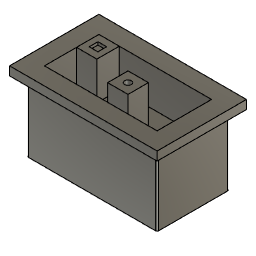
Button_Body (Autodesk Fusion 360 design; units mm, degrees)
Autodesk Fusion 360 part; units mm, degrees
sketch "Sketch1" plane through (0, 0, 0) normal (0, 0, 1) x (1, 0, 0)
  line L0 (0.5, 0) -> (44.2, 0)
  line L1 (44.7, 0.5) -> (44.7, 24.2)
  line L2 (44.2, 24.7) -> (0.5, 24.7)
  line L3 (44.7, 24.7) -> (0, 0) construction
  line L4 (0, 24.7) -> (44.7, 0) construction
  arc A0 (0.5, 24.7) -> (0, 24.2) centre (0.5, 24.2) ccw
  arc A1 (0, 0.5) -> (0.5, 0) centre (0.5, 0.5) ccw
  arc A2 (44.2, 0) -> (44.7, 0.5) centre (44.2, 0.5) ccw
  arc A3 (44.7, 24.2) -> (44.2, 24.7) centre (44.2, 24.2) ccw
  line L5 (22.35, 12.35) -> (22.35, 24.7) construction
  line L6 (22.35, 12.35) -> (0, 12.35) construction
  line L7 (22.35, 12.35) -> (22.35, 0) construction
  circle A4 centre (39.7, 12.35) radius 1.35
  circle A5 centre (5, 12.35) radius 1.35
  line L8 (22.35, 24.7) -> (22.35, 21.7) construction
  line L9 (22.35, 0) -> (22.35, 3) construction
  line L10 (0, 12.35) -> (3, 12.35) construction
  line L11 (3.5, 21.7) -> (41.2, 21.7)
  line L12 (41.2, 3) -> (3.5, 3)
  arc A6 (3.5, 21.7) -> (3, 21.2) centre (3.5, 21.2) ccw
  arc A7 (3, 3.5) -> (3.5, 3) centre (3.5, 3.5) ccw
  arc A8 (41.2, 3) -> (41.7, 3.5) centre (41.2, 3.5) ccw
  arc A9 (41.7, 21.2) -> (41.2, 21.7) centre (41.2, 21.2) ccw
  line L13 (0, 24.2) -> (0, 0.5)
  circle A10 centre (5, 12.35) radius 3
  line L14 (3, 21.2) -> (3, 14.5861)
  line L15 (3, 3.5) -> (3, 10.1139)
  circle A11 centre (39.7, 12.35) radius 3
  line L16 (41.7, 3.5) -> (41.7, 10.1139)
  line L17 (41.7, 21.2) -> (41.7, 14.5861)
  point P0 (22.35, 12.35)
  dimension "d1" = 44.7
  dimension "d2" = 24.7
  dimension "d3" = 0.5
  dimension "d4" = 0.5
  dimension "d5" = 0.5
  dimension "d6" = 0.5
  dimension "d8" = 5
  dimension "d9" = 2.7
  dimension "d10" = 2.7
  dimension "d11" = 3
  dimension "d13" = 0.5
  dimension "d14" = 0.5
  dimension "d15" = 0.5
  dimension "d16" = 0.5
  dimension "d17" = 6
  dimension "d18" = 6
  constraint horizontal L0
  constraint vertical L1
  constraint horizontal L2
  constraint coincident L3.end origin
  constraint midpoint L3 P0
  constraint coincident L4.start L2
  constraint tangent L2 A0
  constraint coincident L3.end L0
  constraint tangent L0 A1
  constraint coincident L4.end L1
  constraint coincident L4.end L0
  constraint tangent L1 A2
  constraint tangent L0 A2
  constraint coincident L3.start L2
  constraint coincident L3.start L1
  constraint tangent L2 A3
  constraint tangent L1 A3
  constraint coincident P0 L5.start
  constraint midpoint L2 L5.end
  constraint midpoint L0 L7.end
  constraint perpendicular L2 L8
  constraint coincident L7 L9.end
  constraint horizontal L11
  constraint horizontal L12
  constraint tangent L11 A6
  constraint tangent L12 A7
  constraint tangent L12 A8
  constraint tangent L11 A9
  constraint tangent A1 L13
  constraint concentric A5 A10
  constraint coincident A10 L14.end
  constraint tangent A6 L14
  constraint vertical L14
  constraint coincident A10 L15.end
  constraint tangent A7 L15
  constraint vertical L15
  constraint concentric A4 A11
  constraint coincident A11 L16.end
  constraint tangent A8 L16
  constraint vertical L16
  constraint coincident A11 L17.end
  constraint tangent A9 L17
  constraint parallel L16 L17
  measures "d1" distance of L3.end L4.end
  measures "d2" distance of L0 L2
  measures "d3" radius of A0
  measures "d4" radius of A1
  measures "d5" radius of A2
  measures "d6" radius of A3
  measures "d8" distance of L6.end A5.centre
  measures "d9" diameter of A4
  measures "d10" diameter of A5
  measures "d11" distance of L5.end L8.end
  measures "d13" radius of A6
  measures "d14" radius of A7
  measures "d15" radius of A8
  measures "d16" radius of A9
  measures "d17" diameter of A10
  measures "d18" diameter of A11
extrude "Extrude1" add sketch "Sketch1" along normal blind 10 contours L0 L1 L2 A0 A1 A2 A3 L13 | A10 | A11 makes body 1
sketch "Sketch3" plane through (0, 0, 10) normal (0, 0, 1) x (-1, 0, 0)
  line L0 (0, -24.2) -> (0, -0.5)
  arc A0 (0, -0.5) -> (-0.5, 0) centre (-0.5, -0.5) ccw
  line L1 (-0.5, 0) -> (-44.2, 0)
  arc A1 (-44.2, 0) -> (-44.7, -0.5) centre (-44.2, -0.5) ccw
  line L2 (-44.7, -0.5) -> (-44.7, -24.2)
  arc A2 (-44.7, -24.2) -> (-44.2, -24.7) centre (-44.2, -24.2) ccw
  line L3 (-44.2, -24.7) -> (-0.5, -24.7)
  arc A3 (-0.5, -24.7) -> (0, -24.2) centre (-0.5, -24.2) ccw
  line L4 (-0.5, 0) -> (-44.2, 0)
  line L5 (-44.7, -0.5) -> (-44.7, -24.2)
  line L6 (-44.2, -24.7) -> (-0.5, -24.7)
  line L7 (0, -24.2) -> (0, -0.5)
  arc A4 (-0.5, -24.7) -> (0, -24.2) centre (-0.5, -24.2) ccw
  arc A5 (0, -0.5) -> (-0.5, 0) centre (-0.5, -0.5) ccw
  arc A6 (-44.2, 0) -> (-44.7, -0.5) centre (-44.2, -0.5) ccw
  arc A7 (-44.7, -24.2) -> (-44.2, -24.7) centre (-44.2, -24.2) ccw
  line L8 (-22.35, -24.7) -> (-22.35, 0) construction
  line L9 (-44.7, -12.35) -> (0, -12.35) construction
  circle A8 centre (-22.35, -12.35) radius 2
  line L10 (-24.35, -12.35) -> (-24.35, 0) construction
  line L11 (-20.35, -12.35) -> (-20.35, -24.7) construction
  line L12 (-20.35, -12.35) -> (-20.35, 0) construction
  line L13 (-24.35, -12.35) -> (-36.35, -12.35) construction
  line L14 (-20.35, -12.35) -> (-8.35, -12.35) construction
  line L15 (-36.35, -12.35) -> (-36.35, -24.7) construction
  line L16 (-36.35, -12.35) -> (-36.35, 0) construction
  line L17 (-8.35, -12.35) -> (-8.35, -24.7) construction
  line L18 (-8.35, -12.35) -> (-8.35, 0) construction
  line L19 (-36.35, -12.35) -> (-36.35, -17.35) construction
  line L20 (-36.35, -12.35) -> (-36.35, -7.35) construction
  line L21 (-36.35, -7.35) -> (-26.35, -7.35) construction
  line L22 (-26.35, -17.35) -> (-36.35, -17.35) construction
  line L23 (-8.35, -7.35) -> (-8.35, -17.3527) construction
  line L24 (-24.35, -12.35) -> (-24.35, -24.7) construction
  line L25 (-24.35, -12.35) -> (-26.35, -12.35)
  line L26 (-26.35, -12.35) -> (-26.35, -17.35) construction
  line L27 (-26.35, -12.35) -> (-26.35, -7.35) construction
  line L28 (-20.35, -12.35) -> (-18.35, -12.35)
  line L29 (-18.35, -12.35) -> (-18.35, -17.3527) construction
  line L30 (-18.35, -17.3527) -> (-8.35, -17.3527) construction
  line L31 (-8.35, -7.35) -> (-18.35, -7.35) construction
  line L32 (-18.35, -7.35) -> (-18.35, -12.35) construction
  line L33 (-36.35, -17.35) -> (-26.35, -7.35) construction
  line L34 (-26.35, -17.35) -> (-36.35, -7.35) construction
  line L35 (-8.35, -17.3527) -> (-18.35, -7.35) construction
  line L36 (-18.35, -17.3527) -> (-8.35, -7.35) construction
  circle A9 centre (-13.35, -12.3513) radius 1
  circle A10 centre (-31.35, -12.35) radius 1
  point P0 (-44.7, 0)
  point P1 (-44.7, -24.7)
  dimension "d21" = 24.7
  dimension "d22" = 0.5
  dimension "d23" = 0.5
  dimension "d24" = 0.5
  dimension "d25" = 0.5
  dimension "d26" = 4
  dimension "d36" = 2
  dimension "d37" = 2
  constraint parallel L1 L4
  constraint perpendicular L4 L5
  constraint perpendicular L5 L6
  constraint perpendicular L4 L7
  constraint tangent L6 A4
  constraint tangent L7 A4
  constraint tangent L4 A5
  constraint tangent L7 A5
  constraint coincident P0 L4
  constraint coincident P0 L5
  constraint tangent L4 A6
  constraint tangent L5 A6
  constraint coincident P1 L5
  constraint coincident P1 L6
  constraint tangent L5 A7
  constraint tangent L6 A7
  constraint midpoint L6 L8.start
  constraint midpoint L4 L8.end
  constraint midpoint L5 L9.start
  constraint midpoint L7 L9.end
  constraint midpoint L9 A8.centre
  constraint coincident A8 L10.start
  constraint coincident L9 L10.start
  constraint coincident L4 L10.end
  constraint tangent A8 L10
  constraint coincident A8 L11.start
  constraint coincident L9 L11.start
  constraint coincident L6 L11.end
  constraint tangent A8 L11
  constraint coincident L4 L12.end
  constraint tangent A8 L12
  constraint horizontal L13
  constraint perpendicular L12 L14
  constraint coincident L6 L15.end
  constraint perpendicular L6 L15
  constraint coincident L4 L16.end
  constraint perpendicular L4 L16
  constraint coincident L6 L17.end
  constraint perpendicular L6 L17
  constraint coincident L4 L18.end
  constraint perpendicular L4 L18
  constraint perpendicular L9 L19
  constraint perpendicular L13 L20
  constraint horizontal L21
  constraint perpendicular L19 L22
  constraint coincident L18 L23.start
  constraint coincident L17 L23.end
  constraint coincident L6 L24.end
  constraint perpendicular L6 L24
  constraint perpendicular L24 L25
  constraint perpendicular L13 L26
  constraint perpendicular L21 L27
  constraint perpendicular L11 L28
  constraint perpendicular L28 L29
  constraint perpendicular L17 L30
  constraint perpendicular L29 L31
  constraint perpendicular L9 L32
  constraint perpendicular L33 L34
  constraint midpoint L36 A9.centre
  constraint midpoint L34 A10.centre
  measures "d21" distance of P0 P1
  measures "d22" radius of A4
  measures "d23" radius of A5
  measures "d24" radius of A6
  measures "d25" radius of A7
  measures "d26" diameter of A8
  measures "d36" diameter of A9
  measures "d37" diameter of A10
extrude "Extrude2" add sketch "Sketch3" along normal blind 4 bodies 1
sketch "Sketch5" plane through (0, 0, 14) normal (0, 0, 1) x (-1, 0, 0)
  circle A0 centre (-13.35, -12.3513) radius 1
  circle A1 centre (-31.35, -12.35) radius 1
  circle A2 centre (-22.35, -12.35) radius 2
  arc A3 (-44.7, -24.2) -> (-44.2, -24.7) centre (-44.2, -24.2) ccw
  line L0 (-44.2, -24.7) -> (-0.5, -24.7)
  arc A4 (-0.5, -24.7) -> (0, -24.2) centre (-0.5, -24.2) ccw
  line L1 (0, -24.2) -> (0, -0.5)
  arc A5 (0, -0.5) -> (-0.5, 0) centre (-0.5, -0.5) ccw
  line L2 (-0.5, 0) -> (-44.2, 0)
  arc A6 (-44.2, 0) -> (-44.7, -0.5) centre (-44.2, -0.5) ccw
  line L3 (-44.7, -0.5) -> (-44.7, -24.2)
  line L4 (0, 0) -> (0, -24.7)
  line L5 (0, -24.7) -> (-44.7, -24.7)
  line L6 (-44.7, -24.7) -> (-44.7, 0)
  line L7 (-44.7, 0) -> (0, 0)
  line L8 (-3, -21.7) -> (-41.7, -21.7)
  line L9 (-41.7, -21.7) -> (-41.7, -3)
  line L10 (-41.7, -3) -> (-3, -3)
  line L11 (-3, -3) -> (-3, -21.7)
  line L12 (-18.85, -12.35) -> (-18.85, -15.85)
  line L13 (-18.85, -15.85) -> (-22.35, -15.85)
  line L14 (-25.85, -15.85) -> (-22.35, -15.85)
  line L15 (-18.85, -12.35) -> (-18.85, -8.85)
  line L16 (-18.85, -8.85) -> (-22.35, -8.85)
  line L17 (-25.85, -8.85) -> (-22.35, -8.85)
  line L18 (-25.85, -15.85) -> (-25.85, -8.85)
  point P0 (-3, -21.7)
  point P1 (-3, -3)
  point P2 (-41.7, -21.7)
  point P3 (-41.7, -3)
  dimension "d40" = 44.7
  constraint coincident L4.start L7.end
  constraint perpendicular L0 L4
  constraint perpendicular L4 L5
  constraint perpendicular L5 L6
  constraint perpendicular L4 L7
  constraint horizontal L8
  constraint vertical L9
  constraint horizontal L10
  constraint vertical L11
  constraint coincident P3 L9.end
  constraint coincident P0 L8.start
  constraint perpendicular L17 L18
  measures "d40" distance of L4.end L5.end
extrude "Extrude3" add sketch "Sketch5" along normal blind 10 contours L12 L13 L14 L15 L16 L17 L18 bodies 1
sketch "Sketch10" plane through (0, 8.85, 0) normal (0, -1, 0) x (1, 0, 0)
  line L0 (18.85, 14) -> (25.85, 14)
  line L1 (25.85, 14) -> (25.85, 24)
  line L2 (25.85, 24) -> (18.85, 24)
  line L3 (18.85, 24) -> (18.85, 14)
  line L4 (22.35, 18) -> (24.35, 18)
  line L5 (24.35, 18) -> (24.35, 14)
  line L6 (22.35, 14) -> (24.35, 14)
  line L7 (22.35, 14) -> (20.35, 14)
  line L8 (20.35, 14) -> (20.35, 18)
  line L9 (20.35, 18) -> (22.35, 18)
  constraint midpoint L0 L6.start
  constraint perpendicular L1 L4
  constraint coincident L0 L5.end
  constraint perpendicular L0 L5
  constraint perpendicular L4 L8
extrude "Extrude4" cut sketch "Sketch10" against normal blind 4 contours L0 L4 L5 L6 L7 L8 L9 bodies 1
sketch "Sketch11" plane through (0, 0, 24) normal (0, 0, 1) x (-1, 0, 0)
  circle A0 centre (-22.35, -12.35) radius 2
  line L0 (-18.85, -15.85) -> (-18.85, -8.85)
  line L1 (-18.85, -8.85) -> (-25.85, -8.85)
  line L2 (-25.85, -8.85) -> (-25.85, -15.85)
  line L3 (-25.85, -15.85) -> (-18.85, -15.85)
  line L4 (-18.85, -15.85) -> (-25.85, -8.85) construction
  line L5 (-25.85, -15.85) -> (-18.85, -8.85) construction
  circle A1 centre (-22.35, -12.35) radius 1.15
  dimension "d58" = 2.3
  constraint coincident L0.start L3.end
  constraint coincident L1.end L2.start
  constraint coincident L2.end L3.start
  constraint coincident L0.end L1.start
  constraint concentric A0 A1
  measures "d58" diameter of A1
extrude "Extrude5" add sketch "Sketch11" against normal blind 8 separate body contours A0 makes body 2
sketch "Sketch12" plane through (0, 0, 14) normal (0, 0, 1) x (-1, 0, 0)
  line L0 (-18.85, -15.85) -> (-25.85, -15.85)
  line L1 (-25.85, -15.85) -> (-25.85, -8.85)
  line L2 (-25.85, -8.85) -> (-24.35, -8.85)
  line L3 (-24.35, -8.85) -> (-24.35, -12.35)
  arc A0 (-20.35, -12.35) -> (-24.35, -12.35) centre (-22.35, -12.35) ccw
  line L4 (-20.35, -12.35) -> (-20.35, -8.85)
  line L5 (-20.35, -8.85) -> (-18.85, -8.85)
  line L6 (-18.85, -8.85) -> (-18.85, -15.85)
  circle A1 centre (-13.35, -12.3513) radius 1
  circle A2 centre (-31.35, -12.35) radius 1
  arc A3 (-44.7, -24.2) -> (-44.2, -24.7) centre (-44.2, -24.2) ccw
  line L7 (-44.2, -24.7) -> (-0.5, -24.7)
  arc A4 (-0.5, -24.7) -> (0, -24.2) centre (-0.5, -24.2) ccw
  line L8 (0, -24.2) -> (0, -0.5)
  arc A5 (0, -0.5) -> (-0.5, 0) centre (-0.5, -0.5) ccw
  line L9 (-0.5, 0) -> (-44.2, 0)
  arc A6 (-44.2, 0) -> (-44.7, -0.5) centre (-44.2, -0.5) ccw
  line L10 (-44.7, -0.5) -> (-44.7, -24.2)
  line L11 (-3, -21.7) -> (-41.7, -21.7)
  line L12 (-41.7, -21.7) -> (-41.7, -3)
  line L13 (-41.7, -3) -> (-3, -3)
  line L14 (-3, -3) -> (-3, -21.7)
  point P0 (-3, -21.7)
  point P1 (-41.7, -21.7)
  point P2 (-41.7, -3)
  point P3 (-3, -3)
  constraint horizontal L11
  constraint vertical L12
  constraint horizontal L13
  constraint vertical L14
  constraint coincident P2 L12.end
  constraint coincident P0 L11.start
extrude "Extrude6" add sketch "Sketch12" along normal blind 10 contours A3 L7 A4 L8 A5 L9 A6 L10 bodies 1
sketch "Sketch14" plane through (0, 0, 24) normal (0, 0, 1) x (-1, 0, 0)
  line L0 (-41.7, -3) -> (-3, -3)
  line L1 (-3, -3) -> (-3, -21.7)
  line L2 (-3, -21.7) -> (-41.7, -21.7)
  line L3 (-41.7, -21.7) -> (-41.7, -3)
  line L4 (-44.7, -0.5) -> (-44.7, -24.2)
  arc A0 (-44.7, -24.2) -> (-44.2, -24.7) centre (-44.2, -24.2) ccw
  line L5 (-44.2, -24.7) -> (-0.5, -24.7)
  arc A1 (-0.5, -24.7) -> (0, -24.2) centre (-0.5, -24.2) ccw
  line L6 (0, -24.2) -> (0, -0.5)
  arc A2 (0, -0.5) -> (-0.5, 0) centre (-0.5, -0.5) ccw
  line L7 (-0.5, 0) -> (-44.2, 0)
  arc A3 (-44.2, 0) -> (-44.7, -0.5) centre (-44.2, -0.5) ccw
  line L8 (3, -27.7) -> (-47.7, -27.7)
  line L9 (-47.7, -27.7) -> (-47.7, 3)
  line L10 (-47.7, 3) -> (3, 3)
  line L11 (3, 3) -> (3, -27.7)
  point P0 (3, -27.7)
  point P1 (3, 3)
  point P2 (-47.7, 3)
  point P3 (-47.7, -27.7)
  constraint horizontal L8
  constraint vertical L9
  constraint horizontal L10
  constraint vertical L11
  constraint coincident P2 L9.end
  constraint coincident P0 L8.start
extrude "Extrude7" add sketch "Sketch14" along normal blind 3 contours L4 A0 L5 A1 L6 A2 L7 A3 | L8 L9 L10 L11 bodies 1
extrude "Extrude8" add 2 faces at (20.6408, 12.4494, 24) (22.3998, 15.3481, 24) along direction (0, 0, 1) blind 3 on bodies 1 2 bodies 2 1
sketch "Sketch15" plane through (0, 0, 14) normal (0, 0, 1) x (-1, 0, 0)
  line L0 (-41.7, -3) -> (-41.7, -21.7)
  line L1 (-41.7, -21.7) -> (-3, -21.7)
  line L2 (-3, -21.7) -> (-3, -3)
  line L3 (-3, -3) -> (-41.7, -3)
  line L4 (-18.85, -15.85) -> (-25.85, -15.85)
  line L5 (-25.85, -15.85) -> (-25.85, -8.85)
  line L6 (-25.85, -8.85) -> (-24.35, -8.85)
  line L7 (-24.35, -8.85) -> (-24.35, -12.35)
  arc A0 (-20.35, -12.35) -> (-24.35, -12.35) centre (-22.35, -12.35) ccw
  line L8 (-20.35, -12.35) -> (-20.35, -8.85)
  line L9 (-20.35, -8.85) -> (-18.85, -8.85)
  line L10 (-18.85, -8.85) -> (-18.85, -15.85)
  circle A1 centre (-13.35, -12.3513) radius 1
  circle A2 centre (-31.35, -12.35) radius 1
  line L11 (-3, -21.7) -> (-10, -21.7)
  line L12 (-10, -21.7) -> (-10, -14)
  line L13 (-10, -14) -> (-3, -14)
  constraint coincident L1.end L2.start
  constraint coincident L1 L11.end
  constraint perpendicular L11 L12
  constraint coincident L2 L13.end
  constraint perpendicular L2 L13
extrude "Extrude9" add sketch "Sketch15" along normal blind 13 separate body contours L1 L2 L11 L12 L13 makes body 3
sketch "Sketch16" plane through (0, 0, 27) normal (0, 0, 1) x (-1, 0, 0)
  line L0 (-3, -21.7) -> (-3, -14)
  line L1 (-3, -14) -> (-10, -14)
  line L2 (-10, -14) -> (-10, -21.7)
  line L3 (-10, -21.7) -> (-3, -21.7)
  line L4 (-6.5, -19.35) -> (-8, -19.35)
  line L5 (-8, -19.35) -> (-8, -16.35)
  line L6 (-8, -16.35) -> (-5, -16.35)
  line L7 (-6.5, -19.35) -> (-5, -19.35)
  line L8 (-5, -19.35) -> (-5, -16.35)
  constraint perpendicular L6 L8
extrude "Extrude10" cut sketch "Sketch16" against normal blind 1 contours L4 L5 L6 L7 L8 bodies 3
